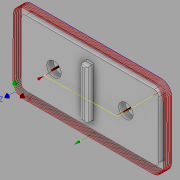
# Autodesk Inventor part: rocker_frame_mount_00
Saved by Autodesk Inventor 2021.3 (Build 253353000, 353)
## iProperties
Created: 2021-07-09
Part Number: rocker_frame_mount_00
Material: Generic
Document SubType Name: Modeling
Designer: gisen
Density: 1 g/cm^3
Appearance: Default
Author: gisen
Autodesk Inventor part; units mm, degrees
ref_plane "YZ Plane" through (0, 0, 0) normal (1, 0, 0) x (0, 1, 0)
ref_plane "XZ Plane" through (0, 0, 0) normal (0, 1, 0) x (-1, 0, 0)
ref_plane "XY Plane" through (0, 0, 0) normal (0, 0, 1) x (1, 0, 0)
sketch "スケッチ2" plane through (0, 0, 0) normal (0, 0, 1) x (1, 0, 0)
  line L0 (-31.5, 15) -> (31.5, 15)
  line L1 (31.5, 15) -> (31.5, -15)
  line L2 (31.5, -15) -> (-31.5, -15)
  line L3 (-31.5, -15) -> (-31.5, 15)
  line L4 (0, 24.6) -> (0, -21.6) construction
  line L5 (-44.1, 0) -> (44.1, 0) construction
  line L6 (-31.5, 15) -> (31.5, 15)
  line L7 (31.5, 15) -> (31.5, 18)
  line L8 (31.5, 18) -> (-31.5, 18)
  line L9 (-31.5, 18) -> (-31.5, 15)
  point P0 (0, 0)
  point P1 (31.5, 15)
  dimension "d1" = 63
  dimension "d2" = 30
  dimension "d3" = 15
  dimension "d4" = 31.5
  dimension "d26" = 3
  constraints: 16 end point, 4 parallel, 2 horizontal, 2 perpendicular
  measures "d1" distance of L1.end L2.end
  measures "d2" distance of L0.end L1.end
  measures "d3" distance between parallel lines of L0 L5
  measures "d4" distance between parallel lines of L4 L3
  measures "d26" distance of L7.end L6.end
extrude "押し出し1" add sketch "スケッチ2" along normal blind 3 contours L0 L1 L2 L3
sketch "スケッチ3" plane through (0, 0, 3) normal (0, 0, 1) x (1, 0, 0)
  line L0 (-31.5, -15) -> (31.5, -15) construction
  line L1 (-44.1, 0) -> (44.1, 0) construction
  line L2 (31.5, -15) -> (31.5, 15) projected
  line L3 (31.5, 15) -> (-31.5, 15) projected
  line L4 (-31.5, 15) -> (-31.5, -15) projected
  point P0 (0, 0)
  point P1 (-16.5, 0)
  point P2 (16.5, 0)
  constraints: 2 point on line
hole "穴1" at (-16.5, 0, 3) at (16.5, 0, 3) direction (0, 0, -1) diameter 6.6 end through all
fillet "フィレット1" radius 2 4 edges at (31.5, -15, 1.5) (-31.5, -15, 1.5) (-31.5, 15, 1.5) (31.5, 15, 1.5)
sketch "スケッチ4" plane through (0, 0, 3) normal (0, 0, 1) x (1, 0, 0)
  line L0 (-29.5, -15) -> (29.5, -15) projected
  arc A0 (-31.5, -13) -> (-29.5, -15) centre (-29.5, -13) ccw projected
  line L1 (-29.5, -15) -> (29.5, -15) projected
  arc A1 (29.5, -15) -> (31.5, -13) centre (29.5, -13) ccw projected
  circle A2 centre (-16.5, 0) radius 3.3 projected
  circle A3 centre (16.5, 0) radius 3.3 projected
  line L2 (1.5, -11) -> (-1.5, -11)
  line L3 (-1.5, -11) -> (-1.5, 11)
  line L4 (-1.5, 11) -> (1.5, 11)
  line L5 (1.5, 11) -> (1.5, -11)
  line L6 (1.5, -11) -> (-1.5, 11) construction
  line L7 (-1.5, -11) -> (1.5, 11) construction
  line L8 (31.5, -13) -> (31.5, 13) projected
  line L9 (29.5, 15) -> (-29.5, 15) projected
  line L10 (-31.5, 13) -> (-31.5, -13) projected
  arc A4 (31.5, 13) -> (29.5, 15) centre (29.5, 13) ccw projected
  arc A5 (-29.5, 15) -> (-31.5, 13) centre (-29.5, 13) ccw projected
  point P0 (0, 0)
  dimension "d22" = 3
  dimension "d24" = 4
  constraints: 12 end point, 2 midpoint, 2 parallel, 1 horizontal, 1 perpendicular
  measures "d22" distance of L3.end L4.end
  measures "d24" distance between parallel lines of L0 L2
extrude "押し出し2" add sketch "スケッチ4" along normal blind 3 contours L2 L3 L4 L5
fillet "フィレット2" radius 1 2 edges at (-1.5, 0, 6) (1.5, 0, 6)
fillet "フィレット2" radius 0.5 4 edges at (0, 11, 3) (0, -11, 3) (0, 11, 6) (0, -11, 6)
equation "\"d3\" = 0.5 * d2"
equation "\"d4\" = 0.5 * d1"
equation "\"d24\" = d23"
equation "\"d23\" = 4"
